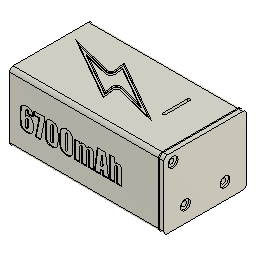
Juicebox (Autodesk Fusion 360 design; units mm, degrees)
Autodesk Fusion 360 part; units mm, degrees
sketch "footprint" plane through (0, 0, 0) normal (0, 0, 1) x (1, 0, 0) in component "IP5328P"
  line L0 (0, 0) -> (65, 0)
  line L1 (65, 0) -> (65, 32.5)
  line L2 (65, 32.5) -> (0, 32.5)
  line L3 (0, 32.5) -> (0, 0)
  line L4 (32.5, 32.5) -> (32.5, 0) construction
  line L5 (65, 16.25) -> (0, 16.25) construction
  line L6 (62.5, 29.75) -> (2.5, 29.75) construction
  line L7 (2.5, 29.75) -> (2.5, 2.75) construction
  line L8 (2.5, 2.75) -> (62.5, 2.75) construction
  line L9 (62.5, 2.75) -> (62.5, 29.75) construction
  line L10 (62.5, 29.75) -> (2.5, 2.75) construction
  line L11 (2.5, 29.75) -> (62.5, 2.75) construction
  circle A0 centre (62.5, 29.75) radius 1.5
  circle A1 centre (62.5, 2.75) radius 1.5
  circle A2 centre (2.5, 2.75) radius 1.5
  circle A3 centre (2.5, 29.75) radius 1.5
  line L12 (8, 32.5) -> (21, 32.5)
  line L13 (21, 32.5) -> (21, 21.5)
  line L14 (21, 21.5) -> (8, 21.5)
  line L15 (8, 21.5) -> (8, 32.5)
  line L16 (28, 32.5) -> (37, 32.5)
  line L17 (37, 32.5) -> (37, 25.5)
  line L18 (37, 25.5) -> (28, 25.5)
  line L19 (28, 25.5) -> (28, 32.5)
  line L20 (44, 32.5) -> (57, 32.5)
  line L21 (57, 32.5) -> (57, 21.5)
  line L22 (57, 21.5) -> (44, 21.5)
  line L23 (44, 21.5) -> (44, 32.5)
  line L24 (0, 7) -> (7, 7)
  line L25 (7, 7) -> (7, 15)
  line L26 (7, 15) -> (0, 15)
  line L27 (0, 15) -> (0, 7)
  line L28 (0, 21) -> (4, 21)
  line L29 (4, 21) -> (4, 26)
  line L30 (4, 26) -> (0, 26)
  line L31 (0, 26) -> (0, 21)
  line L32 (1, 21) -> (1, 26)
  line L33 (62.5, 8.75) -> (64, 8.75) construction
  line L34 (64, 8.75) -> (64, 23.75) construction
  line L35 (64, 23.75) -> (62.5, 23.75)
  line L36 (62.5, 23.75) -> (62.5, 8.75)
  line L37 (62.5, 23) -> (62.5, 9.5)
  arc A4 (62.5, 9.5) -> (64, 9.5) centre (63.25, 9.5) ccw
  line L38 (64, 9.5) -> (64, 23)
  arc A5 (64, 23) -> (62.5, 23) centre (63.25, 23) ccw
  line L39 (63.25, 23.75) -> (63.25, 8.75) construction
  point P0 (32.5, 16.25)
  dimension "d1" = 65
  dimension "d2" = 32.5
  dimension "d5" = 60
  dimension "d6" = 27
  dimension "d7" = 3
  dimension "d8" = 3
  dimension "d9" = 3
  dimension "d10" = 3
  dimension "d11" = 13
  dimension "d12" = 11
  dimension "d13" = 8
  dimension "d14" = 9
  dimension "d15" = 7
  dimension "d16" = 7
  dimension "d17" = 8
  dimension "d27" = 7
  dimension "d28" = 8
  dimension "d29" = 7
  dimension "d30" = 4
  dimension "d31" = 5
  dimension "d32" = 6
  dimension "d179" = 3
  dimension "d212" = 15
  dimension "d213" = 1.5
  constraint horizontal L0
  constraint vertical L1
  constraint horizontal L2
  constraint vertical L3
  constraint coincident L0.start L3.end
  constraint midpoint L2 L4.start
  constraint perpendicular L2 L4
  constraint midpoint L1 L5.start
  constraint midpoint L3 L5.end
  constraint horizontal L6
  constraint perpendicular L6 L7
  constraint parallel L6 L8
  constraint parallel L7 L9
  constraint coincident L10 P0
  constraint coincident L11 P0
  constraint midpoint L5 P0
  constraint coincident L6.start L9.end
  constraint coincident L8.end L9.start
  constraint coincident L7.end L8.start
  constraint coincident L6.end L7.start
  constraint horizontal L12
  constraint vertical L13
  constraint horizontal L14
  constraint vertical L15
  constraint coincident L2 L12.start
  constraint horizontal L16
  constraint vertical L17
  constraint horizontal L18
  constraint vertical L19
  constraint coincident L2 L16.start
  constraint horizontal L20
  constraint vertical L21
  constraint horizontal L22
  constraint vertical L23
  constraint coincident L2 L20.start
  constraint equal L14 L22
  constraint equal L13 L23
  constraint horizontal L24
  constraint vertical L25
  constraint horizontal L26
  constraint vertical L27
  constraint coincident L3 L24.start
  constraint horizontal L28
  constraint vertical L29
  constraint horizontal L30
  constraint vertical L31
  constraint coincident L3 L28.start
  constraint coincident L28 L32.start
  constraint coincident L30 L32.end
  constraint perpendicular L30 L32
  constraint horizontal L33
  constraint vertical L34
  constraint horizontal L35
  constraint vertical L36
  constraint coincident L9 L33.start
  constraint midpoint L9 L36
  constraint tangent L37 A4
  constraint tangent A4 L38
  constraint parallel L37 L38
  constraint tangent L38 A5
  constraint tangent L37 A5
  constraint midpoint A5 L39.start
  constraint midpoint A4 L39.end
  constraint midpoint L33 L39.end
  constraint perpendicular L33 L39
  constraint midpoint L35 L39.start
  measures "d1" distance of L0.start L0.end
  measures "d2" distance of L0.start L2.end
  measures "d5" distance of L7.end L8.end
  measures "d6" distance of L6.end L7.end
  measures "d7" diameter of A0
  measures "d8" diameter of A1
  measures "d9" diameter of A2
  measures "d10" diameter of A3
  measures "d11" distance of L12.start L12.end
  measures "d12" distance of L12.start L14.end
  measures "d13" distance of L3 L15
  measures "d14" distance of L16.start L16.end
  measures "d15" distance of L16.start L18.end
  measures "d16" distance of L13 L19
  measures "d17" distance of L1 L21
  measures "d27" distance of L24.start L24.end
  measures "d28" distance of L24.start L26.end
  measures "d29" distance of L0 L24
  measures "d30" distance of L28.start L28.end
  measures "d31" distance of L28.start L30.end
  measures "d32" distance of L26 L28
  measures "d179" distance of L29 L32
  measures "d212" distance of L33 L35
  measures "d213" distance of L33.start L33.end
extrude "Extrude1" add sketch "footprint" along normal blind 1.6 contours L0 L1 L2 L3 L13 L14 L15 L17 L18 L19 L21 L22 L23 L24 L25 L26 L28 L29 L30 | L3 L24 L25 L26 L27 | L3 L28 L30 L31 L32 | L28 L29 L30 L32 | L2 L16 L17 L18 L19 | L35 L36 A5 | L36 L37 A4 L38 A5 makes body 1 in component "IP5328P"
extrude "Extrude2" add sketch "footprint" along normal blind 6 separate body contours L2 L20 L21 L22 L23 | L2 L12 L13 L14 L15 makes body 2 at (12.3333, 28.8333, 0) makes body 3 at (48.3333, 28.8333, 0) in component "IP5328P"
extrude "Extrude3" add sketch "footprint" along normal blind 4 from surface at 1.6 separate body contours L2 L16 L17 L18 L19 makes body 4 in component "IP5328P"
sketch "ports_front" plane through (0, 32.5, 0) normal (0, 1, 0) x (-1, 0, 0) in component "IP5328P"
  line L0 (-57, 0) -> (-44, 0)
  line L1 (-44, 0) -> (-44, 6)
  line L2 (-44, 6) -> (-57, 6)
  line L3 (-57, 6) -> (-57, 0)
  line L4 (-21, 0) -> (-8, 0)
  line L5 (-8, 0) -> (-8, 6)
  line L6 (-8, 6) -> (-21, 6)
  line L7 (-21, 6) -> (-21, 0)
  line L8 (-37, 1.6) -> (-28, 1.6)
  line L9 (-28, 1.6) -> (-28, 5.6)
  line L10 (-28, 5.6) -> (-37, 5.6)
  line L11 (-37, 5.6) -> (-37, 1.6)
  line L12 (-35, 1.6) -> (-30, 1.6)
  arc A0 (-30, 1.6) -> (-30, 5.6) centre (-30, 3.6) ccw
  line L13 (-30, 5.6) -> (-35, 5.6)
  arc A1 (-35, 5.6) -> (-35, 1.6) centre (-35, 3.6) ccw
  line L14 (-37, 3.6) -> (-28, 3.6) construction
  line L15 (-44, 1.6) -> (-21, 1.6)
  line L16 (-25, 1.6) -> (-24, 1.6)
  line L17 (-24, 1.6) -> (-24, 2.6)
  line L18 (-24, 2.6) -> (-25, 2.6)
  line L19 (-25, 2.6) -> (-25, 1.6)
  line L20 (-21, 1.6) -> (-28, 1.6) construction
  dimension "d214" = 1
  dimension "d215" = 1
  constraint tangent L12 A0
  constraint tangent A0 L13
  constraint parallel L12 L13
  constraint tangent L13 A1
  constraint tangent L12 A1
  constraint midpoint A1 L14.start
  constraint midpoint A0 L14.end
  constraint midpoint L9 L14.end
  constraint perpendicular L9 L14
  constraint midpoint L11 L14.start
  constraint collinear L10 L13
  constraint horizontal L16
  constraint vertical L17
  constraint horizontal L18
  constraint vertical L19
  constraint coincident L15 L16.start
  constraint coincident L15.end L20.start
  constraint coincident L8.end L9.start
  constraint midpoint L16 L20
  measures "d214" distance of L16.start L16.end
  measures "d215" distance of L16.start L18.end
extrude "Extrude4" cut sketch "ports_front" against normal up to surface (7 mm away) contours L8 L10 L12 A0 L13 A1 L15 keep common part bodies 4 in component "IP5328P"
extrude "Extrude5" add sketch "footprint" along normal blind 3 from surface at 1.6 separate body contours L3 L24 L25 L26 L27 makes body 5 in component "IP5328P"
extrude "Extrude6" add sketch "footprint" along normal blind 3.2 from surface at 1.6 separate body contours L3 L28 L30 L31 L32 | L28 L29 L30 L32 makes body 6 in component "IP5328P"
sketch "ports_side" plane through (0, 0, 0) normal (-1, 0, 0) x (0, -1, 0) in component "IP5328P"
  line L0 (-26, 1.6) -> (-21, 1.6)
  line L1 (-21, 1.6) -> (-21, 4.8)
  line L2 (-21, 4.8) -> (-26, 4.8)
  line L3 (-26, 4.8) -> (-26, 1.6)
  circle A0 centre (-23.5, 3.2) radius 1
  line L4 (-26, 3.2) -> (-21, 3.2) construction
  line L5 (-23.5, 4.8) -> (-23.5, 1.6) construction
  line L6 (-15, 1.6) -> (-7, 1.6)
  line L7 (-7, 1.6) -> (-7, 4.6)
  line L8 (-7, 4.6) -> (-15, 4.6)
  line L9 (-15, 4.6) -> (-15, 1.6)
  line L10 (-15, 4.6) -> (-7, 4.6)
  line L11 (-15, 4.6) -> (-15, 3.4)
  line L12 (-14, 1.6) -> (-8, 1.6)
  line L13 (-14, 1.6) -> (-15, 3.4)
  line L14 (-7, 4.6) -> (-7, 3.4)
  line L15 (-15, 4.6) -> (-15, 3.4)
  line L16 (-7, 3.4) -> (-8, 1.6)
  dimension "d39" = 2
  dimension "d42" = 1.2
  dimension "d43" = 6
  constraint midpoint L3 L4.start
  constraint midpoint L1 L4.end
  constraint midpoint L2 L5.start
  constraint midpoint L0 L5.end
  constraint midpoint A0.centre L4
  constraint coincident L8 L9.start
  constraint coincident L7.end L8.start
  constraint perpendicular L7 L10
  constraint coincident L8.end L9.start
  constraint perpendicular L10 L11
  constraint coincident L6 L12.start
  constraint perpendicular L9 L12
  constraint midpoint L6 L12
  constraint coincident L7 L14.end
  constraint equal L14 L15
  measures "d39" diameter of A0
  measures "d42" distance of L8.end L11.end
  measures "d43" distance of L12.start L12.end
extrude "Extrude7" cut sketch "ports_side" against normal blind 1 contours L0 L1 L2 L3 bodies 6 in component "IP5328P"
extrude "Extrude8" cut sketch "ports_side" against normal blind 7 contours L6 L7 L8 L9 L10 L11 L12 L13 L14 L15 L16 keep common part bodies 5 in component "IP5328P"
sketch "Bottom_Screws" plane through (0, 0, 0) normal (0, 0, 1) x (1, 0, 0) in component "Battery_Holder"
  line L0 (0, -9.5) -> (80, -9.5)
  line L1 (80, -9.5) -> (80, 32.5)
  line L2 (80, 32.5) -> (0, 32.5)
  line L3 (0, 32.5) -> (0, -9.5)
  line L4 (40, -9.5) -> (40, 32.5) construction
  line L5 (80, 11.5) -> (0, 11.5) construction
  line L6 (12, 1.5) -> (68, 1.5) construction
  line L7 (68, 1.5) -> (68, 21.5) construction
  line L8 (68, 21.5) -> (12, 21.5) construction
  line L9 (12, 21.5) -> (12, 1.5) construction
  line L10 (12, 1.5) -> (68, 21.5) construction
  line L11 (68, 1.5) -> (12, 21.5) construction
  circle A0 centre (68, 1.5) radius 1.5
  circle A1 centre (12, 1.5) radius 1.5
  circle A2 centre (12, 21.5) radius 1.5
  circle A3 centre (68, 21.5) radius 1.5
  line L12 (0, 0) -> (65, 0)
  line L13 (65, 0) -> (65, 32.5)
  line L14 (0, 32.5) -> (0, 0)
  line L15 (65, 32.5) -> (0, 32.5)
  point P0 (40, 11.5)
  point P1 (0, 32.5)
  dimension "d46" = 80
  dimension "d47" = 42
  dimension "d48" = 56
  dimension "d49" = 20
  dimension "d50" = 3
  dimension "d51" = 3
  dimension "d52" = 3
  dimension "d53" = 3
  constraint horizontal L0
  constraint vertical L1
  constraint horizontal L2
  constraint vertical L3
  constraint midpoint L0 L4.start
  constraint midpoint L2 L4.end
  constraint midpoint L1 L5.start
  constraint midpoint L3 L5.end
  constraint horizontal L6
  constraint perpendicular L6 L7
  constraint parallel L6 L8
  constraint parallel L7 L9
  constraint coincident L10 P0
  constraint coincident L11 P0
  constraint midpoint L5 P0
  constraint coincident L6.end L7.start
  constraint coincident L6.start L9.end
  constraint coincident L8.end L9.start
  constraint coincident L7.end L8.start
  constraint coincident P1 L2.end
  measures "d46" distance of L0.start L0.end
  measures "d47" distance of L0.start L2.end
  measures "d48" distance of L7.end L8.end
  measures "d49" distance of L6.end L7.end
  measures "d50" diameter of A0
  measures "d51" diameter of A1
  measures "d52" diameter of A2
  measures "d53" diameter of A3
extrude "Extrude1'" add sketch "Bottom_Screws" against normal blind 22 from surface at -2 separate body makes body 7 in component "Battery_Holder"
sketch "Side_screws" plane through (80, 0, 0) normal (1, 0, 0) x (0, 1, 0) in component "Battery_Holder"
  line L0 (32.5, -2) -> (-9.5, -2)
  line L1 (-9.5, -2) -> (-9.5, -24)
  line L2 (-9.5, -24) -> (32.5, -24)
  line L3 (32.5, -24) -> (32.5, -2)
  line L4 (22.5, -24) -> (22.5, -19) construction
  line L5 (32.5, -19) -> (22.5, -19) construction
  line L6 (11.5, -2) -> (11.5, -24)
  circle A0 centre (22.5, -19) radius 1.25
  circle A1 centre (0.5, -19) radius 1.25
  line L7 (-9.5, -19) -> (0.5, -19) construction
  line L8 (0.5, -24) -> (0.5, -19) construction
  dimension "d152" = 5
  dimension "d153" = 10
  dimension "d154" = 2.5
  constraint coincident L2 L4.start
  constraint vertical L4
  constraint coincident L3 L5.start
  constraint horizontal L5
  constraint midpoint L0 L6.start
  constraint midpoint L2 L6.end
  constraint coincident L4.end L5.end
  constraint symmetric L4.start L6 L8.start
  constraint symmetric L4.end L6 A1.centre
  constraint symmetric L5.start L6 L7.start
  constraint symmetric L6 A0 A1
  measures "d152" distance of L4.start L4.end
  measures "d153" distance of L4.end L5.start
  measures "d154" diameter of A0
sketch "Midplate" plane through (0, 0, -2) normal (0, 0, 1) x (-1, 0, 0) in component "Enclosure"
  circle A0 centre (-68, -1.5) radius 1.5
  circle A1 centre (-68, -21.5) radius 1.5
  circle A2 centre (-12, -1.5) radius 1.5
  circle A3 centre (-12, -21.5) radius 1.5
  line L0 (-80, -32.5) -> (0, -32.5)
  line L1 (0, -32.5) -> (0, 9.5)
  line L2 (0, 9.5) -> (-80, 9.5)
  line L3 (-80, 9.5) -> (-80, -32.5)
  circle A4 centre (-2.5, -2.75) radius 1.5
  circle A5 centre (-2.5, -29.75) radius 1.5
  circle A6 centre (-62.5, -2.75) radius 1.5
  circle A7 centre (-62.5, -29.75) radius 1.5
  circle A8 centre (-68, -21.5) radius 1.5
  circle A9 centre (-68, -1.5) radius 1.5
  circle A10 centre (-12, -21.5) radius 1.5
  circle A11 centre (-12, -1.5) radius 1.5
  line L4 (-12, -21.5) -> (-68, -21.5) construction
  line L5 (-12, -1.5) -> (-12, -21.5) construction
  line L6 (-2.5, -29.75) -> (-2.5, -2.75) construction
  line L7 (-62.5, -29.75) -> (-62.5, -2.75) construction
  line L8 (-12, -21.5) -> (-2.5, -29.75) construction
  line L9 (-12, -1.5) -> (-2.5, -2.75) construction
  line L10 (-62.5, -2.75) -> (-68, -1.5) construction
  line L11 (-62.5, -2.75) -> (-12, -1.5) construction
  line L12 (-12.1305, -2.4915) -> (-3.5, -3.627)
  line L13 (-3.5, -27.5571) -> (-3.5, -3.627)
  line L14 (-11.6264, -20.5) -> (-3.5, -27.5571)
  line L15 (-11.6264, -20.5) -> (-68, -20.5)
  line L16 (-11.8695, -0.5085) -> (-1.5, -1.873)
  line L17 (-1.5, -31.9429) -> (-1.5, -1.873)
  line L18 (-12.3736, -22.5) -> (-1.5, -31.9429)
  line L19 (-12.3736, -22.5) -> (-68, -22.5)
  line L20 (-61.5, -29.75) -> (-61.5, -1.9518)
  line L21 (-61.5, -1.9518) -> (-67.7784, -0.5249)
  line L22 (-63.5, -29.75) -> (-63.5, -3.5482)
  line L23 (-63.5, -3.5482) -> (-68.2216, -2.4751)
  line L24 (-62.4753, -3.7497) -> (-13, -2.5251)
  line L25 (-13, -2.5251) -> (-13, -21.5)
  line L26 (-62.5247, -1.7503) -> (-11, -0.4749)
  line L27 (-11, -0.4749) -> (-11, -21.5)
  circle A12 centre (-62.5, -29.75) radius 2.5
  circle A13 centre (-68, -21.5) radius 2.5
  circle A14 centre (-68, -1.5) radius 2.5
  circle A15 centre (-62.5, -2.75) radius 2.5
  circle A16 centre (-12, -1.5) radius 2.5
  circle A17 centre (-2.5, -2.75) radius 2.5
  circle A18 centre (-2.5, -29.75) radius 2.5
  circle A19 centre (-12, -21.5) radius 2.5
  dimension "d193" = 1
  dimension "d194" = -1
  dimension "d195" = 1
  dimension "d196" = -1
  dimension "d197" = 1
  dimension "d198" = -1
  dimension "d199" = 1
  dimension "d200" = 1
  dimension "d201" = 1
  dimension "d202" = 1
  dimension "d203" = 1
  dimension "d204" = 1
  dimension "d205" = 1
  dimension "d206" = 1
  constraint coincident A3.centre A10.centre
  constraint coincident A1.centre A8.centre
  constraint coincident A6.centre L7.end
  constraint coincident A2.centre A11.centre
  constraint coincident A5.centre L6.start
  constraint coincident A7.centre L7.start
  constraint coincident A4.centre L6.end
  constraint coincident A0.centre A9.centre
extrude "Extrude23" add sketch "Midplate" along normal up to surface (2 mm away) separate body contours A0 A9 L21 L23 A14 | A0 A9 L21 L23 A14 | L21 L23 A14 A15 | A6 L21 L26 A15 | A6 L21 L23 A15 | A6 L22 L23 A15 | A6 L24 L26 A15 | L24 L26 A15 A16 | L15 L20 L22 A15 | A6 L20 L22 A15 | A2 A11 L16 L26 A16 | A2 A11 L24 L26 A16 | L15 L19 L22 A13 | L15 L19 L20 L22 | A6 L20 L24 A15 | A2 A11 L12 L16 L27 A16 | L12 L16 A16 A17 | A2 A11 L24 L25 A16 | L15 L19 L20 A19 | A1 A8 L15 L19 A13 | A1 A8 L15 L19 A13 | L19 L20 L22 A12 | A4 L16 L17 A17 | A4 L12 L16 A17 | L25 L27 A16 A19 | A2 A11 L12 L25 L27 A16 | A3 A10 L15 L25 A19 | A3 A10 L15 L19 A19 | A7 L20 L22 A12 | A7 L20 L22 A12 | A4 L12 L13 A17 | L12 L27 A16 | A3 A10 L25 L27 A19 | A3 A10 L18 L19 A19 | A5 L17 L18 A18 | A4 L13 L17 A17 | L13 L17 A17 A18 | A3 A10 L14 L27 A19 | L14 L18 A18 A19 | A3 A10 L14 L18 A19 | A5 L13 L14 L17 L18 A18 | A5 L17 L18 picked at (-1.7525, -31.3892) makes body 8 in component "Enclosure"
sketch "Shell_frame" plane through (80, 0, 0) normal (1, 0, 0) x (0, 1, 0) in component "Enclosure"
  line L0 (32.5, -2) -> (-9.5, -2)
  line L1 (-9.5, -2) -> (-9.5, -24)
  line L2 (-9.5, -24) -> (32.5, -24)
  line L3 (32.5, -24) -> (32.5, -2)
  line L4 (21.5, 0) -> (32.5, 0)
  line L5 (32.5, 0) -> (32.5, 6)
  line L6 (32.5, 6) -> (21.5, 6)
  line L7 (21.5, 6) -> (21.5, 0)
  line L8 (-11.5, 10) -> (34.5, 10)
  line L9 (34.5, 10) -> (34.5, -28)
  line L10 (34.5, -28) -> (-11.5, -28)
  line L11 (-11.5, -28) -> (-11.5, 10)
  line L12 (-9.5, -26) -> (32.5, -26)
  line L13 (32.5, -26) -> (32.5, 8)
  line L14 (32.5, 8) -> (-9.5, 8)
  line L15 (-9.5, 8) -> (-9.5, -26)
  line L16 (-10.3, 8.8) -> (33.3, 8.8)
  line L17 (33.3, 8.8) -> (33.3, -26.8)
  line L18 (33.3, -26.8) -> (-10.3, -26.8)
  line L19 (-10.3, -26.8) -> (-10.3, 8.8)
  line L20 (-10.7, 9.2) -> (33.7, 9.2)
  line L21 (33.7, 9.2) -> (33.7, -27.2)
  line L22 (33.7, -27.2) -> (-10.7, -27.2)
  line L23 (-10.7, -27.2) -> (-10.7, 9.2)
  line L24 (-4.3682, 9.2) -> (-4.3682, 5)
  line L25 (-6.3682, 3) -> (-10.7, 3)
  arc A0 (-6.3682, 3) -> (-4.3682, 5) centre (-6.3682, 5) ccw
  circle A1 centre (-6.3682, 5) radius 1.25
  dimension "d129" = 2
  dimension "d130" = 2
  dimension "d131" = 4
  dimension "d132" = 4
  dimension "d133" = 2
  dimension "d134" = 2
  dimension "d135" = 1.2
  dimension "d136" = 0.8
  dimension "d155" = 2
  dimension "d156" = 2.5
  constraint horizontal L8
  constraint vertical L9
  constraint horizontal L10
  constraint vertical L11
  constraint horizontal L12
  constraint vertical L13
  constraint horizontal L14
  constraint vertical L15
  constraint collinear L1 L15
  constraint collinear L3 L13
  constraint coincident L20 L24.start
  constraint perpendicular L14 L24
  constraint coincident L23 L25.end
  constraint perpendicular L23 L25
  constraint tangent L24 A0
  constraint tangent L25 A0
  constraint concentric A0 A1
  measures "d129" distance of L1 L11
  measures "d130" distance of L3 L9
  measures "d131" distance of L6 L8
  measures "d132" distance of L2 L10
  measures "d133" distance of L8 L14
  measures "d134" distance of L10 L12
  measures "d155" radius of A0
  measures "d156" diameter of A1
extrude "Extrude12" add sketch "Shell_frame" against normal up to surface (80 mm away) separate body contours L1 L3 L5 L12 L13 L14 L15 L16 L17 L18 L19 L24 L25 | L14 L15 L16 L19 L24 L25 | L16 L19 L20 L23 L24 L25 | L16 L17 L18 L19 L20 L21 L22 L23 L24 L25 | L8 L9 L10 L11 makes body 9 in component "Enclosure"
extrude "Extrude13" add sketch "Shell_frame" against normal blind 2 from surface at -80 contours L0 L1 L2 L3 L13 L15 | L1 L3 L5 L12 L13 L14 L15 L16 L17 L18 L19 L24 L25 | L0 L4 L6 L7 L13 L14 L15 L24 L25 A0 | L2 L12 L13 L15 | L4 L5 L6 L7 L13 | L14 L15 L16 L19 L24 L25 | L14 L15 L24 L25 A0 | L16 L19 L20 L23 L24 L25 | L16 L17 L18 L19 L20 L21 L22 L23 L24 L25 | L8 L9 L10 L11 | A1 bodies 9 in component "Enclosure"
extrude "Extrude14" cut sketch "ports_front" along normal up to surface (2 mm away) contours L0 L1 L2 L3 | L4 L5 L6 L7 | L8 L10 L12 A0 L13 A1 L15 | L15 L16 L17 L18 L19 bodies 9 in component "Enclosure"
extrude "Extrude19" add sketch "Shell_frame" against normal blind 2 contours L14 L15 L24 L25 A0 bodies 9 in component "Enclosure"
extrude "Extrude15" cut sketch "ports_side" along normal up to surface (2 mm away) contours L0 L1 L2 L3 | A0 | L6 L7 L8 L9 L10 L11 L12 L13 L14 L15 L16 bodies 9 in component "Enclosure"
extrude "Extrude24" cut sketch "footprint" along normal through all contours L36 L37 A4 L38 A5 bodies 9 in component "Enclosure"
extrude "Extrude16" add sketch "Shell_frame" along normal blind 4 separate body contours L0 L1 L2 L3 L13 L15 | L1 L3 L5 L12 L13 L14 L15 L16 L17 L18 L19 L24 L25 | L0 L4 L6 L7 L13 L14 L15 L24 L25 A0 | L2 L12 L13 L15 | L4 L5 L6 L7 L13 | L14 L15 L16 L19 L24 L25 | L14 L15 L24 L25 A0 | L16 L19 L20 L23 L24 L25 | L16 L17 L18 L19 L20 L21 L22 L23 L24 L25 | L8 L9 L10 L11 | A1 makes body 10 in component "Enclosure"
extrude "Extrude18" cut sketch "Shell_frame" along normal blind 1.6 contours L16 L19 L20 L23 L24 L25 | L16 L17 L18 L19 L20 L21 L22 L23 L24 L25 | L8 L9 L10 L11 bodies 10 in component "Enclosure"
extrude "Extrude17" add sketch "Shell_frame" along normal blind 1 contours L8 L9 L10 L11 bodies 9 in component "Enclosure"
sketch "Screw_bores" plane through (84, 0, 0) normal (1, 0, 0) x (0, 1, 0) in component "Enclosure"
  line L0 (-11.5, -28) -> (34.5, -28)
  line L1 (34.5, -28) -> (34.5, 10)
  line L2 (34.5, 10) -> (-11.5, 10)
  line L3 (-11.5, 10) -> (-11.5, -28)
  circle A0 centre (-6.3682, 5) radius 1.25
  circle A1 centre (0.5, -19) radius 1.25
  circle A2 centre (22.5, -19) radius 1.25
hole "Hole2" at (84, -6.3682, 5) at (84, 0.5, -19) at (84, 22.5, -19) direction (-1, 0, 0) diameter 2.7 depth 8 tip angle 180 counterbore diameter 5.5 counterbore depth 0.9 bodies 7 in component "Battery_Holder"
hole "Hole2'" at (84, -6.3682, 5) at (84, 0.5, -19) at (84, 22.5, -19) direction (-1, 0, 0) diameter 2.7 depth 8 tip angle 180 counterbore diameter 5.5 counterbore depth 0.9 bodies 9 10 in component "Enclosure"
sketch "Screw_bores_back" plane through (-2, 0, 0) normal (-1, 0, 0) x (0, -1, 0) in component "Enclosure"
  line L0 (-8, 1.6) -> (-14, 1.6)
  line L1 (-14, 1.6) -> (-15, 3.4)
  line L2 (-15, 3.4) -> (-15, 4.6)
  line L3 (-15, 4.6) -> (-7, 4.6)
  line L4 (-7, 4.6) -> (-7, 3.4)
  line L5 (-7, 3.4) -> (-8, 1.6)
  line L6 (-21, 1.6) -> (-26, 1.6)
  line L7 (-26, 1.6) -> (-26, 4.8)
  line L8 (-26, 4.8) -> (-21, 4.8)
  line L9 (-21, 4.8) -> (-21, 1.6)
  line L10 (-34.5, 10) -> (-34.5, -28)
  line L11 (-34.5, -28) -> (11.5, -28)
  line L12 (11.5, -28) -> (11.5, 10)
  line L13 (11.5, 10) -> (-34.5, 10)
  circle A0 centre (-22.5, -19) radius 1.25
  circle A1 centre (-0.5, -19) radius 1.25
  circle A2 centre (-23.5, 3.2) radius 1
  line L14 (-21.4, 2) -> (-24.6465, 2)
  line L15 (-24.6465, 2) -> (-24.6465, 4.4)
  line L16 (-24.6465, 4.4) -> (-21.4, 4.4)
  line L17 (-21.4, 4.4) -> (-21.4, 2)
  line L18 (-24.6465, 3.9131) -> (-26, 3.9131)
  line L19 (-24.6465, 3.2) -> (-26, 3.2)
  line L20 (-24.6465, 2.4869) -> (-26, 2.4869)
  dimension "d180" = 0.4
  dimension "d181" = 0.4
  dimension "d182" = 0.4
  constraint horizontal L14
  constraint vertical L15
  constraint horizontal L16
  constraint vertical L17
  constraint coincident L15 L18.start
  constraint coincident L7 L18.end
  constraint perpendicular L7 L18
  constraint midpoint L15 L19.start
  constraint perpendicular L15 L19
  constraint symmetric L18.start L19 L20.start
  constraint symmetric L18.end L19 L20.end
  measures "d180" distance of L8 L16
  measures "d181" distance of L6 L14
  measures "d182" distance of L9 L17
hole "Hole3" at (-2, 22.5, -19) at (-2, 0.5, -19) direction (1, 0, 0) diameter 2.9 depth 8 tip angle 180 counterbore diameter 5.5 counterbore depth 0.9 bodies 7 in component "Battery_Holder"
hole "Hole3'" at (-2, 22.5, -19) at (-2, 0.5, -19) direction (1, 0, 0) diameter 2.9 depth 8 tip angle 180 counterbore diameter 5.5 counterbore depth 0.9 bodies 9 in component "Enclosure"
extrude "Extrude22" add sketch "Screw_bores_back" along normal blind 1 from surface at -2 contours L7 L15 L19 L20 | L7 L15 L18 L19 bodies 9 in component "Enclosure"
extrude "Extrude20" add sketch "Screw_bores_back" against normal up to surface (2 mm away) contours L14 L15 L16 L17 | A2 bodies 9 in component "Enclosure"
fillet "Fillet2" radius 2 20 edges at (39.5, 34.5, 10) (39.5, 34.5, -28) (39.5, -11.5, 10) (39.5, -11.5, -28) (39, -9.5, 8) (40, 32.5, 8) (40, 32.5, -26) (40, -9.5, -26) (80.5, -10.7, 9.2) (80.5, 33.7, 9.2) (80.5, 33.7, -27.2) (80.5, -10.7, -27.2) (82.8, -11.5, -28) (82.8, -11.5, 10) (82.8, 34.5, 10) (82.8, 34.5, -28) (80.8, 33.3, 8.8) (80.8, -10.3, 8.8) (80.8, 33.3, -26.8) (80.8, -10.3, -26.8) on bodies 9 10 in component "Enclosure"
sketch "Decal_Lightning" plane through (0, 0, 10) normal (0, 0, 1) x (-1, 0, 0) in component "Enclosure"
  line L0 (-62.5, -9.5) -> (-62.5, -23)
  arc A0 (-64, -23) -> (-62.5, -23) centre (-63.25, -23) ccw
  line L1 (-64, -23) -> (-64, -9.5)
  arc A1 (-62.5, -9.5) -> (-64, -9.5) centre (-63.25, -9.5) ccw
  line L2 (2, 9.5) -> (-81, 9.5)
  line L3 (-81, 9.5) -> (-81, -32.5)
  line L4 (-81, -32.5) -> (2, -32.5)
  line L5 (2, -32.5) -> (2, 9.5)
  line L6 (-53.5185, -6.3923) -> (-34.6599, -17.1603)
  line L7 (-29.448, -20.1363) -> (-30.1485, -15.2325)
  line L8 (-27.4209, -12.7912) -> (-12.6317, -16.6077)
  line L9 (-12.6317, -16.6077) -> (-31.4904, -5.8397)
  line L10 (-36.7022, -2.8637) -> (-36.0017, -7.7675)
  line L11 (-38.7293, -10.2088) -> (-53.5185, -6.3923)
  line L12 (-33.0751, -32.5) -> (-33.0751, 9.5) construction
  line L13 (-30.615, -11.9669) -> (-31.4904, -5.8397) construction
  line L14 (-35.5352, -11.0331) -> (-34.6599, -17.1603) construction
  line L15 (-34.6599, -17.1603) -> (-29.448, -20.1363)
  line L16 (-31.4904, -5.8397) -> (-36.7022, -2.8637)
  line L17 (-34.0963, -4.3517) -> (-32.0539, -18.6483) construction
  line L18 (-5.6515, -19.4419) -> (-30.9945, -4.9713)
  line L19 (-30.9945, -4.9713) -> (-37.9812, -0.9819)
  line L20 (-37.9812, -0.9819) -> (-37.2037, -6.4245)
  line L21 (-39.9313, -8.8659) -> (-60.4987, -3.5581)
  line L22 (-60.4987, -3.5581) -> (-35.1557, -18.0287)
  line L23 (-35.1557, -18.0287) -> (-28.169, -22.0181)
  line L24 (-28.169, -22.0181) -> (-28.9465, -16.5755)
  line L25 (-26.2189, -14.1341) -> (-5.6515, -19.4419)
  arc A2 (-39.9313, -8.8659) -> (-37.2037, -6.4245) centre (-39.3816, -6.7356) ccw
  arc A3 (-26.2189, -14.1341) -> (-28.9465, -16.5755) centre (-26.7686, -16.2644) ccw
  arc A4 (-27.4209, -12.7912) -> (-30.1485, -15.2325) centre (-27.9706, -14.9214) ccw
  arc A5 (-38.7293, -10.2088) -> (-36.0017, -7.7675) centre (-38.1796, -8.0786) ccw
  dimension "d218" = 2.2
  constraint parallel L6 L9
  constraint parallel L7 L10
  constraint parallel L8 L11
  constraint parallel L7 L13
  constraint parallel L10 L14
  constraint parallel L9 L15
  constraint parallel L6 L16
  constraint midpoint L16 L17.start
  constraint midpoint L15 L17.end
  constraint midpoint L12 L17
  constraint coincident L4 L12.start
  constraint coincident L2 L12.end
  constraint tangent L20 A2
  constraint tangent L21 A2
  constraint tangent L24 A3
  constraint tangent L25 A3
  constraint equal A2 A3
  constraint coincident L13.start L7
  constraint coincident L13.start L8
  constraint tangent L7 A4
  constraint tangent L8 A4
  constraint equal A2 A4
  constraint coincident L14.start L11
  constraint coincident L14.start L10
  constraint tangent L11 A5
  constraint tangent L10 A5
  constraint equal A2 A5
  measures "d218" radius of A2
extrude "Extrude25" cut sketch "Decal_Lightning" against normal blind 0.6 contours L18 L19 L20 L21 L22 L23 L24 L25 A2 A3 bodies 9 in component "Enclosure"
extrude "Extrude26" cut sketch "Decal_Lightning" along normal blind 0.6 from surface at -38 contours L18 L19 L20 L21 L22 L23 L24 L25 A2 A3 bodies 9 in component "Enclosure"
chamfer "Chamfer1" distance 0.4 angle 45 32 edges at (37.9144, 8.3749, -28) (50.215, 6.212, -28) (37.5925, 3.7032, -28) (44.3339, 12.7881, -27.4) (28.2359, 14.6251, -28) (15.9352, 16.788, -28) (28.5578, 19.2968, -28) (21.8164, 10.2119, -28) (20.0263, 14.6995, -28) (29.4379, 13.2821, -28) (29.7983, 17.6844, -28) (24.667, 9.7357, -28) (36.7124, 9.7179, -28) (36.352, 5.3156, -28) (46.1239, 8.3005, -28) (41.4832, 13.2643, -28) (44.3339, 12.7881, 10) (28.5578, 19.2968, 10) (15.9352, 16.788, 10) (28.2359, 14.6251, 10) (21.8164, 10.2119, 10) (37.9144, 8.3749, 10) (37.5925, 3.7032, 10) (50.215, 6.212, 10) (36.352, 5.3156, 10) (36.7124, 9.7179, 10) (46.1239, 8.3005, 10) (24.667, 9.7357, 10) (29.7983, 17.6844, 10) (29.4379, 13.2821, 10) (20.0263, 14.6995, 10) (41.4832, 13.2643, 10) on bodies 9 in component "Enclosure"
sketch "Capacity" plane through (0, -11.5, 0) normal (0, -1, 0) x (1, 0, 0) in component "Enclosure"
  line L0 (-2, -26) -> (-2, 8)
  line L1 (11.1896, -7.1872) -> (8.1952, -7.1872)
  spline S0 degree 2 poles (8.1952, -7.1872) (8.1952, -6.3496) (8.1767, -6.1309) knots 0 0 0 1 1 1
  spline S1 degree 2 poles (8.1767, -6.1309) (8.1581, -5.9123) (7.9988, -5.7641) knots 0 0 0 1 1 1
  spline S2 degree 2 poles (7.9988, -5.7641) (7.8394, -5.6158) (7.5652, -5.6158) knots 0 0 0 1 1 1
  spline S3 degree 2 poles (7.5652, -5.6158) (7.3354, -5.6158) (7.1872, -5.7566) knots 0 0 0 1 1 1
  spline S4 degree 2 poles (7.1872, -5.7566) (7.0389, -5.8975) (7.0167, -6.1198) knots 0 0 0 1 1 1
  spline S5 degree 2 poles (7.0167, -6.1198) (6.9944, -6.3422) (6.9944, -7.0167) knots 0 0 0 1 1 1
  line L2 (6.9944, -7.0167) -> (6.9944, -8.929)
  spline S6 degree 2 poles (6.9944, -8.929) (7.2242, -8.4472) (7.6689, -8.2063) knots 0 0 0 1 1 1
  spline S7 degree 2 poles (7.6689, -8.2063) (8.1137, -7.9654) (8.7659, -7.9654) knots 0 0 0 1 1 1
  spline S8 degree 2 poles (8.7659, -7.9654) (9.5886, -7.9654) (10.2187, -8.4101) knots 0 0 0 1 1 1
  spline S9 degree 2 poles (10.2187, -8.4101) (10.8487, -8.8548) (11.0191, -9.4775) knots 0 0 0 1 1 1
  spline S10 degree 2 poles (11.0191, -9.4775) (11.1896, -10.1001) (11.1896, -11.16) knots 0 0 0 1 1 1
  line L3 (11.1896, -11.16) -> (11.1896, -12.1161)
  spline S11 degree 2 poles (11.1896, -12.1161) (11.1896, -13.3762) (11.0933, -13.9914) knots 0 0 0 1 1 1
  spline S12 degree 2 poles (11.0933, -13.9914) (10.9969, -14.6065) (10.5781, -15.1291) knots 0 0 0 1 1 1
  spline S13 degree 2 poles (10.5781, -15.1291) (10.1594, -15.6516) (9.4293, -15.9407) knots 0 0 0 1 1 1
  spline S14 degree 2 poles (9.4293, -15.9407) (8.6992, -16.2298) (7.7282, -16.2298) knots 0 0 0 1 1 1
  spline S15 degree 2 poles (7.7282, -16.2298) (6.5201, -16.2298) (5.7492, -15.8962) knots 0 0 0 1 1 1
  spline S16 degree 2 poles (5.7492, -15.8962) (4.9784, -15.5627) (4.5596, -14.9364) knots 0 0 0 1 1 1
  spline S17 degree 2 poles (4.5596, -14.9364) (4.1408, -14.3101) (4.0704, -13.6208) knots 0 0 0 1 1 1
  spline S18 degree 2 poles (4.0704, -13.6208) (4, -12.9314) (4, -10.945) knots 0 0 0 1 1 1
  line L4 (4, -10.945) -> (4, -9.2847)
  spline S19 degree 2 poles (4, -9.2847) (4, -7.1427) (4.063, -6.42) knots 0 0 0 1 1 1
  spline S20 degree 2 poles (4.063, -6.42) (4.126, -5.6973) (4.5781, -5.0525) knots 0 0 0 1 1 1
  spline S21 degree 2 poles (4.5781, -5.0525) (5.0303, -4.4077) (5.8122, -4.0852) knots 0 0 0 1 1 1
  spline S22 degree 2 poles (5.8122, -4.0852) (6.5942, -3.7628) (7.617, -3.7628) knots 0 0 0 1 1 1
  spline S23 degree 2 poles (7.617, -3.7628) (8.8771, -3.7628) (9.685, -4.1705) knots 0 0 0 1 1 1
  spline S24 degree 2 poles (9.685, -4.1705) (10.4929, -4.5781) (10.8413, -5.3193) knots 0 0 0 1 1 1
  spline S25 degree 2 poles (10.8413, -5.3193) (11.1896, -6.0605) (11.1896, -7.1872) knots 0 0 0 1 1 1
  spline S26 degree 2 poles (8.1952, -10.9302) (8.1952, -10.2928) (8.0544, -10.0556) knots 0 0 0 1 1 1
  spline S27 degree 2 poles (8.0544, -10.0556) (7.9135, -9.8184) (7.5948, -9.8184) knots 0 0 0 1 1 1
  spline S28 degree 2 poles (7.5948, -9.8184) (7.2835, -9.8184) (7.139, -10.0445) knots 0 0 0 1 1 1
  spline S29 degree 2 poles (7.139, -10.0445) (6.9944, -10.2705) (6.9944, -10.9302) knots 0 0 0 1 1 1
  line L5 (6.9944, -10.9302) -> (6.9944, -13.1019)
  spline S30 degree 2 poles (6.9944, -13.1019) (6.9944, -13.895) (7.1316, -14.1396) knots 0 0 0 1 1 1
  spline S31 degree 2 poles (7.1316, -14.1396) (7.2687, -14.3842) (7.5874, -14.3842) knots 0 0 0 1 1 1
  spline S32 degree 2 poles (7.5874, -14.3842) (7.7801, -14.3842) (7.9876, -14.1952) knots 0 0 0 1 1 1
  spline S33 degree 2 poles (7.9876, -14.1952) (8.1952, -14.0062) (8.1952, -13.176) knots 0 0 0 1 1 1
  line L6 (8.1952, -13.176) -> (8.1952, -10.9302)
  line L7 (17.2971, -4) -> (17.2971, -6.6146)
  line L8 (17.2971, -6.6146) -> (15.3848, -16)
  line L9 (15.3848, -16) -> (12.4052, -16)
  line L10 (12.4052, -16) -> (14.5361, -6.1569)
  line L11 (14.5361, -6.1569) -> (11.575, -6.1569)
  line L12 (11.575, -6.1569) -> (11.575, -4)
  line L13 (11.575, -4) -> (17.2971, -4)
  line L14 (25.0278, -8.0618) -> (25.0278, -12.0642)
  spline S34 degree 2 poles (25.0278, -12.0642) (25.0278, -13.428) (24.8796, -14.0506) knots 0 0 0 1 1 1
  spline S35 degree 2 poles (24.8796, -14.0506) (24.7313, -14.6733) (24.2644, -15.2143) knots 0 0 0 1 1 1
  spline S36 degree 2 poles (24.2644, -15.2143) (23.7974, -15.7554) (23.1377, -15.9926) knots 0 0 0 1 1 1
  spline S37 degree 2 poles (23.1377, -15.9926) (22.4781, -16.2298) (21.6628, -16.2298) knots 0 0 0 1 1 1
  spline S38 degree 2 poles (21.6628, -16.2298) (20.588, -16.2298) (19.8765, -15.9815) knots 0 0 0 1 1 1
  spline S39 degree 2 poles (19.8765, -15.9815) (19.1649, -15.7332) (18.7424, -15.2069) knots 0 0 0 1 1 1
  spline S40 degree 2 poles (18.7424, -15.2069) (18.32, -14.6807) (18.1421, -14.0988) knots 0 0 0 1 1 1
  spline S41 degree 2 poles (18.1421, -14.0988) (17.9642, -13.517) (17.9642, -12.2495) knots 0 0 0 1 1 1
  line L15 (17.9642, -12.2495) -> (17.9642, -8.0618)
  spline S42 degree 2 poles (17.9642, -8.0618) (17.9642, -6.4089) (18.2495, -5.5862) knots 0 0 0 1 1 1
  spline S43 degree 2 poles (18.2495, -5.5862) (18.5349, -4.7634) (19.3836, -4.2668) knots 0 0 0 1 1 1
  spline S44 degree 2 poles (19.3836, -4.2668) (20.2322, -3.7702) (21.4404, -3.7702) knots 0 0 0 1 1 1
  spline S45 degree 2 poles (21.4404, -3.7702) (22.4262, -3.7702) (23.2044, -4.1149) knots 0 0 0 1 1 1
  spline S46 degree 2 poles (23.2044, -4.1149) (23.9827, -4.4595) (24.3681, -4.9561) knots 0 0 0 1 1 1
  spline S47 degree 2 poles (24.3681, -4.9561) (24.7536, -5.4527) (24.8907, -6.0754) knots 0 0 0 1 1 1
  spline S48 degree 2 poles (24.8907, -6.0754) (25.0278, -6.698) (25.0278, -8.0618) knots 0 0 0 1 1 1
  spline S49 degree 2 poles (22.0334, -7.0537) (22.0334, -6.0976) (21.9407, -5.8567) knots 0 0 0 1 1 1
  spline S50 degree 2 poles (21.9407, -5.8567) (21.8481, -5.6158) (21.5071, -5.6158) knots 0 0 0 1 1 1
  spline S51 degree 2 poles (21.5071, -5.6158) (21.1736, -5.6158) (21.0661, -5.8715) knots 0 0 0 1 1 1
  spline S52 degree 2 poles (21.0661, -5.8715) (20.9586, -6.1272) (20.9586, -7.0537) knots 0 0 0 1 1 1
  line L16 (20.9586, -7.0537) -> (20.9586, -12.9092)
  spline S53 degree 2 poles (20.9586, -12.9092) (20.9586, -13.9543) (21.0587, -14.1692) knots 0 0 0 1 1 1
  spline S54 degree 2 poles (21.0587, -14.1692) (21.1587, -14.3842) (21.4923, -14.3842) knots 0 0 0 1 1 1
  spline S55 degree 2 poles (21.4923, -14.3842) (21.8258, -14.3842) (21.9296, -14.1322) knots 0 0 0 1 1 1
  spline S56 degree 2 poles (21.9296, -14.1322) (22.0334, -13.8802) (22.0334, -12.9981) knots 0 0 0 1 1 1
  line L17 (22.0334, -12.9981) -> (22.0334, -7.0537)
  line L18 (33.1662, -8.0618) -> (33.1662, -12.0642)
  spline S57 degree 2 poles (33.1662, -12.0642) (33.1662, -13.428) (33.0179, -14.0506) knots 0 0 0 1 1 1
  spline S58 degree 2 poles (33.0179, -14.0506) (32.8697, -14.6733) (32.4027, -15.2143) knots 0 0 0 1 1 1
  spline S59 degree 2 poles (32.4027, -15.2143) (31.9358, -15.7554) (31.2761, -15.9926) knots 0 0 0 1 1 1
  spline S60 degree 2 poles (31.2761, -15.9926) (30.6164, -16.2298) (29.8011, -16.2298) knots 0 0 0 1 1 1
  spline S61 degree 2 poles (29.8011, -16.2298) (28.7264, -16.2298) (28.0148, -15.9815) knots 0 0 0 1 1 1
  spline S62 degree 2 poles (28.0148, -15.9815) (27.3033, -15.7332) (26.8808, -15.2069) knots 0 0 0 1 1 1
  spline S63 degree 2 poles (26.8808, -15.2069) (26.4583, -14.6807) (26.2804, -14.0988) knots 0 0 0 1 1 1
  spline S64 degree 2 poles (26.2804, -14.0988) (26.1025, -13.517) (26.1025, -12.2495) knots 0 0 0 1 1 1
  line L19 (26.1025, -12.2495) -> (26.1025, -8.0618)
  spline S65 degree 2 poles (26.1025, -8.0618) (26.1025, -6.4089) (26.3879, -5.5862) knots 0 0 0 1 1 1
  spline S66 degree 2 poles (26.3879, -5.5862) (26.6733, -4.7634) (27.5219, -4.2668) knots 0 0 0 1 1 1
  spline S67 degree 2 poles (27.5219, -4.2668) (28.3706, -3.7702) (29.5788, -3.7702) knots 0 0 0 1 1 1
  spline S68 degree 2 poles (29.5788, -3.7702) (30.5645, -3.7702) (31.3428, -4.1149) knots 0 0 0 1 1 1
  spline S69 degree 2 poles (31.3428, -4.1149) (32.1211, -4.4595) (32.5065, -4.9561) knots 0 0 0 1 1 1
  spline S70 degree 2 poles (32.5065, -4.9561) (32.8919, -5.4527) (33.029, -6.0754) knots 0 0 0 1 1 1
  spline S71 degree 2 poles (33.029, -6.0754) (33.1662, -6.698) (33.1662, -8.0618) knots 0 0 0 1 1 1
  spline S72 degree 2 poles (30.1717, -7.0537) (30.1717, -6.0976) (30.0791, -5.8567) knots 0 0 0 1 1 1
  spline S73 degree 2 poles (30.0791, -5.8567) (29.9864, -5.6158) (29.6455, -5.6158) knots 0 0 0 1 1 1
  spline S74 degree 2 poles (29.6455, -5.6158) (29.3119, -5.6158) (29.2044, -5.8715) knots 0 0 0 1 1 1
  spline S75 degree 2 poles (29.2044, -5.8715) (29.097, -6.1272) (29.097, -7.0537) knots 0 0 0 1 1 1
  line L20 (29.097, -7.0537) -> (29.097, -12.9092)
  spline S76 degree 2 poles (29.097, -12.9092) (29.097, -13.9543) (29.197, -14.1692) knots 0 0 0 1 1 1
  spline S77 degree 2 poles (29.197, -14.1692) (29.2971, -14.3842) (29.6306, -14.3842) knots 0 0 0 1 1 1
  spline S78 degree 2 poles (29.6306, -14.3842) (29.9642, -14.3842) (30.0679, -14.1322) knots 0 0 0 1 1 1
  spline S79 degree 2 poles (30.0679, -14.1322) (30.1717, -13.8802) (30.1717, -12.9981) knots 0 0 0 1 1 1
  line L21 (30.1717, -12.9981) -> (30.1717, -7.0537)
  line L22 (37.1983, -6.1643) -> (37.1464, -7.1001)
  spline S80 degree 2 poles (37.1464, -7.1001) (37.4948, -6.5432) (37.9765, -6.2648) knots 0 0 0 1 1 1
  spline S81 degree 2 poles (37.9765, -6.2648) (38.4583, -5.9864) (39.0735, -5.9864) knots 0 0 0 1 1 1
  spline S82 degree 2 poles (39.0735, -5.9864) (40.2742, -5.9864) (40.9636, -7.1001) knots 0 0 0 1 1 1
  spline S83 degree 2 poles (40.9636, -7.1001) (41.3416, -6.5432) (41.8159, -6.2648) knots 0 0 0 1 1 1
  spline S84 degree 2 poles (41.8159, -6.2648) (42.2903, -5.9864) (42.8684, -5.9864) knots 0 0 0 1 1 1
  spline S85 degree 2 poles (42.8684, -5.9864) (43.6319, -5.9864) (44.1322, -6.357) knots 0 0 0 1 1 1
  spline S86 degree 2 poles (44.1322, -6.357) (44.6325, -6.7276) (44.7733, -7.265) knots 0 0 0 1 1 1
  spline S87 degree 2 poles (44.7733, -7.265) (44.9141, -7.8023) (44.9141, -9.0105) knots 0 0 0 1 1 1
  line L23 (44.9141, -9.0105) -> (44.9141, -16)
  line L24 (44.9141, -16) -> (42.0086, -16)
  line L25 (42.0086, -16) -> (42.0086, -9.5886)
  spline S88 degree 2 poles (42.0086, -9.5886) (42.0086, -8.3286) (41.9234, -8.0284) knots 0 0 0 1 1 1
  spline S89 degree 2 poles (41.9234, -8.0284) (41.8382, -7.7282) (41.5269, -7.7282) knots 0 0 0 1 1 1
  spline S90 degree 2 poles (41.5269, -7.7282) (41.2082, -7.7282) (41.1155, -8.0247) knots 0 0 0 1 1 1
  spline S91 degree 2 poles (41.1155, -8.0247) (41.0229, -8.3212) (41.0229, -9.5886) knots 0 0 0 1 1 1
  line L26 (41.0229, -9.5886) -> (41.0229, -16)
  line L27 (41.0229, -16) -> (38.1174, -16)
  line L28 (38.1174, -16) -> (38.1174, -9.7517)
  spline S92 degree 2 poles (38.1174, -9.7517) (38.1174, -8.3064) (38.0469, -8.0173) knots 0 0 0 1 1 1
  spline S93 degree 2 poles (38.0469, -8.0173) (37.9765, -7.7282) (37.6578, -7.7282) knots 0 0 0 1 1 1
  spline S94 degree 2 poles (37.6578, -7.7282) (37.4577, -7.7282) (37.3169, -7.8802) knots 0 0 0 1 1 1
  spline S95 degree 2 poles (37.3169, -7.8802) (37.176, -8.0321) (37.1612, -8.2508) knots 0 0 0 1 1 1
  spline S96 degree 2 poles (37.1612, -8.2508) (37.1464, -8.4694) (37.1464, -9.181) knots 0 0 0 1 1 1
  line L29 (37.1464, -9.181) -> (37.1464, -16)
  line L30 (37.1464, -16) -> (34.2409, -16)
  line L31 (34.2409, -16) -> (34.2409, -6.1643)
  line L32 (34.2409, -6.1643) -> (37.1983, -6.1643)
  line L33 (51.4274, -4) -> (53.2119, -16)
  line L34 (53.2119, -16) -> (50.0229, -16)
  line L35 (50.0229, -16) -> (49.8554, -13.8431)
  line L36 (49.8554, -13.8431) -> (48.7392, -13.8431)
  line L37 (48.7392, -13.8431) -> (48.5516, -16)
  line L38 (48.5516, -16) -> (45.3255, -16)
  line L39 (45.3255, -16) -> (46.9172, -4)
  line L40 (46.9172, -4) -> (51.4274, -4)
  spline S97 degree 2 poles (49.7736, -11.7159) (49.5368, -9.6771) (49.2983, -6.6757) knots 0 0 0 1 1 1
  spline S98 degree 2 poles (49.2983, -6.6757) (48.8215, -10.1224) (48.6995, -11.7159) knots 0 0 0 1 1 1
  line L41 (48.6995, -11.7159) -> (49.7736, -11.7159)
  line L42 (56.6473, -4) -> (56.6473, -6.6998)
  spline S99 degree 2 poles (56.6473, -6.6998) (57.0327, -6.3431) (57.4812, -6.1648) knots 0 0 0 1 1 1
  spline S100 degree 2 poles (57.4812, -6.1648) (57.9296, -5.9864) (58.441, -5.9864) knots 0 0 0 1 1 1
  spline S101 degree 2 poles (58.441, -5.9864) (59.2267, -5.9864) (59.7789, -6.3867) knots 0 0 0 1 1 1
  spline S102 degree 2 poles (59.7789, -6.3867) (60.3311, -6.7869) (60.4534, -7.3094) knots 0 0 0 1 1 1
  spline S103 degree 2 poles (60.4534, -7.3094) (60.5757, -7.832) (60.5757, -9.218) knots 0 0 0 1 1 1
  line L43 (60.5757, -9.218) -> (60.5757, -16)
  line L44 (60.5757, -16) -> (57.5812, -16)
  line L45 (57.5812, -16) -> (57.5812, -9.0772)
  spline S104 degree 2 poles (57.5812, -9.0772) (57.5812, -8.2174) (57.496, -7.9728) knots 0 0 0 1 1 1
  spline S105 degree 2 poles (57.496, -7.9728) (57.4108, -7.7282) (57.1143, -7.7282) knots 0 0 0 1 1 1
  spline S106 degree 2 poles (57.1143, -7.7282) (56.84, -7.7282) (56.7437, -7.9802) knots 0 0 0 1 1 1
  spline S107 degree 2 poles (56.7437, -7.9802) (56.6473, -8.2322) (56.6473, -8.9809) knots 0 0 0 1 1 1
  line L46 (56.6473, -8.9809) -> (56.6473, -16)
  line L47 (56.6473, -16) -> (53.6529, -16)
  line L48 (53.6529, -16) -> (53.6529, -4)
  line L49 (53.6529, -4) -> (56.6473, -4)
extrude "Extrude27" cut sketch "Capacity" against normal blind 0.4 bodies 9 in component "Enclosure"
component "IP5328P" placed x (1, 0, 0) y (0, 1, 0) z (0, 0, 1) at (0, 0, 0)
component "Battery_Holder" placed x (1, 0, 0) y (0, 1, 0) z (0, 0, 1) at (0, 0, 0)
component "Enclosure" placed x (1, 0, 0) y (0, 1, 0) z (0, 0, 1) at (0, 0, 0)
equation "d130 = d129"
equation "d131 = d129 + 2 mm"
equation "d132 = d129 + 2 mm"
equation "d133 = d129"
equation "d134 = d129"
named bodies: "PCB", "USBA_2", "USBA_1", "USBC", "microUSB", "Button", "Case_shell", "Case_cover", "Midplate"
